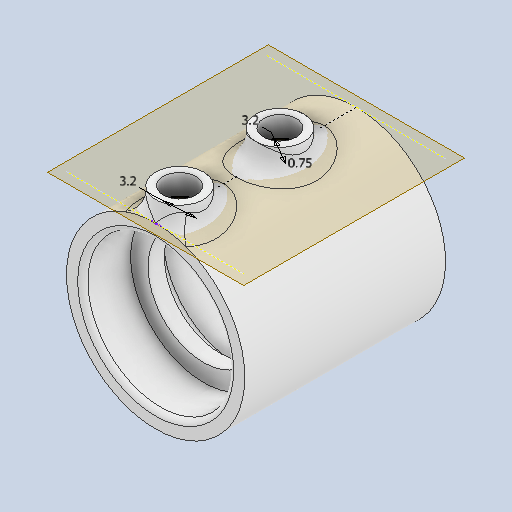
# Autodesk Inventor part: SpectrocameraAdapter12mm
Saved by Autodesk Inventor 2023 (Build 270158000, 158)
## iProperties
Created: 2022-09-02
Part Number: SpectrocameraAdapter12mm
Material: ABS Plastic
Document SubType Name: Modeling
Designer: Miner
Density: 1.06 g/cm^3
Appearance: Smooth - White
Author: Miner
Autodesk Inventor part; units mm, degrees
ref_plane "YZ Plane" through (0, 0, 0) normal (1, 0, 0) x (0, 1, 0)
ref_plane "XY Plane" through (0, 0, 0) normal (0, 0, 1) x (1, 0, 0)
sketch "Sketch1" plane through (0, 0, 0) normal (0, 0, 1) x (1, 0, 0)
  circle A0 centre (0, 0) radius 7.15
  circle A1 centre (0, 0) radius 8.75
  dimension "d0" = 14.3
  dimension "d1" = 1.6
  constraints: 2 centre point, 1 coincident
  measures "d0" diameter of A0
  measures "d1" radial gap between concentric circles of A0 A1
extrude "Extrusion1" add sketch "Sketch1" along normal blind 4.7 and the other way blind 15
sketch "Sketch2" plane through (0, 0, 0) normal (0, 0, 1) x (1, 0, 0)
  circle A0 centre (0, 0) radius 8.65
  circle A1 centre (0, 0) radius 5.45
  dimension "d4" = 3.2
  constraints: 2 centre point, 1 coincident
  measures "d4" radial gap between concentric circles of A0 A1
extrude "Extrusion2" add sketch "Sketch2" against normal blind 1.6
chamfer "Chamfer1" distance 1.6 angle 45 1 edges at (-7.15, 0, -1.6)
ref_plane "Work Plane1" through (0, 8.75, 0) normal (0, 1, 0) x (-1, 0, 0)
sketch "Sketch3" plane through (0, 8.75, 0) normal (0, 1, 0) x (-1, 0, 0)
  line L0 (0, 0) -> (0, 4.7) construction
  line L1 (8.75, 4.7) -> (-8.75, 4.7) construction
  line L2 (0, 0) -> (0, -15) construction
  line L3 (-8.75, -15) -> (8.75, -15) construction
  circle A0 centre (0, 2.35) radius 1.6
  circle A1 centre (0, 2.35) radius 2.35
  circle A2 centre (0, -7.5) radius 1.6
  circle A3 centre (0, -7.5) radius 2.35
  dimension "d13" = 3.2
  dimension "d14" = 3.2
  dimension "d15" = 0.75
  constraints: 4 centre point, 4 end point, 4 midpoint
  measures "d13" diameter of A0
  measures "d14" diameter of A2
  measures "d15" radial gap between concentric circles of A2 A3
extrude "Extrusion3" add sketch "Sketch3" along normal blind 2 and the other way blind 0.5 contours A3
extrude "Extrusion4" add sketch "Sketch3" along normal blind 2 and the other way blind 0.5 contours A1
extrude "Extrusion5" cut sketch "Sketch3" against normal blind 2 contours A0 | A2
fillet "Fillet2" radius 2 3 edges at (-1.7878, 8.5654, -5.9747) (-1.7833, 8.5664, -9.0305) (2.35, 8.4285, -7.5008)
fillet "Fillet3" radius 2 3 edges at (2.35, 8.4285, 2.3492) (-1.7833, 8.5664, 0.8195) (-1.7878, 8.5654, 3.8753)
fillet "Fillet4" radius 0.5 1 edges at (-7.15, 0, 4.7)
fillet "Fillet5" radius 0.5 1 edges at (-7.15, 0, -15)
body "Solid1"
